Autodesk Fusion 360 part; units mm, degrees
note: some values were not read from the file. Set by a fixed rule: which sketch regions a step uses.
(part 18 of 59)
  spline S101 degree 5 poles (29.3284, 22.5421) (29.3257, 22.5422) (29.3203, 22.5423) (29.3122, 22.5425) (29.3014, 22.5428) (29.288, 22.5431) (29.2745, 22.5434) (29.2612, 22.5437) (29.2478, 22.544) (29.2345, 22.5442) (29.2212, 22.5445) (29.2079, 22.5447) (29.1947, 22.5449) (29.1815, 22.5451) (29.1683, 22.5453) (29.1551, 22.5454) (29.142, 22.5455) (29.129, 22.5457) (29.1159, 22.5458) (29.1029, 22.5458) (29.0899, 22.5459) (29.077, 22.546) (29.0641, 22.546) (29.0512, 22.546) (29.0383, 22.546) (29.0255, 22.546) (29.0127, 22.546) (29, 22.5459) (28.9872, 22.5458) (28.9745, 22.5458) (28.9619, 22.5457) (28.9493, 22.5456) (28.9367, 22.5454) (28.9241, 22.5453) (28.9116, 22.5451) (28.8991, 22.5449) (28.8867, 22.5448) (28.8743, 22.5445) (28.8619, 22.5443) (28.8495, 22.5441) (28.8372, 22.5438) (28.8249, 22.5436) (28.8127, 22.5433) (28.8005, 22.543) (28.7883, 22.5427) (28.7762, 22.5423) (28.7641, 22.542) (28.752, 22.5416) (28.74, 22.5412) (28.728, 22.5409) (28.716, 22.5405) (28.7041, 22.54) (28.6922, 22.5396) (28.6803, 22.5392) (28.6685, 22.5387) (28.6567, 22.5382) (28.645, 22.5377) (28.6333, 22.5372) (28.6216, 22.5367) (28.61, 22.5362) (28.5984, 22.5356) (28.5868, 22.5351) (28.5753, 22.5345) (28.5638, 22.5339) (28.5524, 22.5333) (28.541, 22.5327) (28.5296, 22.5321) (28.5183, 22.5314) (28.507, 22.5308) (28.4957, 22.5301) (28.4845, 22.5294) (28.4733, 22.5287) (28.4622, 22.528) (28.4511, 22.5273) (28.44, 22.5266) (28.429, 22.5258) (28.4181, 22.5251) (28.4071, 22.5243) (28.3962, 22.5235) (28.3854, 22.5227) (28.3745, 22.5219) (28.3638, 22.5211) (28.353, 22.5203) (28.3423, 22.5195) (28.3317, 22.5186) (28.321, 22.5177) (28.3105, 22.5169) (28.2999, 22.516) (28.2894, 22.5151) (28.279, 22.5142) (28.2686, 22.5133) (28.2582, 22.5123) (28.2479, 22.5114) (28.2376, 22.5104) (28.2274, 22.5095) (28.2172, 22.5085) (28.207, 22.5075) (28.1969, 22.5065) (28.1868, 22.5055) (28.1768, 22.5045) (28.1668, 22.5035) (28.1569, 22.5025) (28.147, 22.5014) (28.1372, 22.5004) (28.1274, 22.4993) (28.1176, 22.4983) (28.1079, 22.4972) (28.0982, 22.4961) (28.0886, 22.495) (28.079, 22.4939) (28.0695, 22.4928) (28.06, 22.4916) (28.0506, 22.4905) (28.0412, 22.4894) (28.0318, 22.4882) (28.0225, 22.4871) (28.0133, 22.4859) (28.004, 22.4847) (27.9949, 22.4836) (27.9858, 22.4824) (27.9767, 22.4812) (27.9677, 22.48) (27.9587, 22.4788) (27.9498, 22.4776) (27.9409, 22.4763) (27.9321, 22.4751) (27.9233, 22.4739) (27.9146, 22.4726) (27.9059, 22.4714) (27.8973, 22.4701) (27.8887, 22.4689) (27.8802, 22.4676) (27.8717, 22.4664) (27.8633, 22.4651) (27.8549, 22.4638) (27.8466, 22.4625) (27.8383, 22.4612) (27.8301, 22.4599) (27.8219, 22.4586) (27.8138, 22.4573) (27.8057, 22.456) (27.7977, 22.4547) (27.7898, 22.4534) (27.7819, 22.4521) (27.774, 22.4508) (27.7662, 22.4494) (27.7585, 22.4481) (27.7508, 22.4468) (27.7431, 22.4454) (27.7356, 22.4441) (27.728, 22.4428) (27.7206, 22.4414) (27.7132, 22.4401) (27.7058, 22.4387) (27.6985, 22.4374) (27.6912, 22.436) (27.6841, 22.4347) (27.6769, 22.4333) (27.6698, 22.432) (27.6628, 22.4306) (27.6559, 22.4293) (27.649, 22.4279) (27.6421, 22.4266) (27.6353, 22.4252) (27.6286, 22.4239) (27.622, 22.4225) (27.6154, 22.4212) (27.6088, 22.4199) (27.6023, 22.4185) (27.5959, 22.4172) (27.5896, 22.4158) (27.5833, 22.4145) (27.577, 22.4132) (27.5709, 22.4118) (27.5647, 22.4105) (27.5587, 22.4092) (27.5527, 22.4079) (27.5468, 22.4065) (27.5409, 22.4052) (27.5352, 22.4039) (27.5294, 22.4026) (27.5238, 22.4013) (27.5182, 22.4) (27.5127, 22.3987) (27.5072, 22.3974) (27.5018, 22.3962) (27.4965, 22.3949) (27.4912, 22.3936) (27.4861, 22.3924) (27.481, 22.3911) (27.4759, 22.3899) (27.4709, 22.3887) (27.466, 22.3874) (27.4612, 22.3862) (27.4564, 22.385) (27.4517, 22.3838) (27.4471, 22.3827) (27.4426, 22.3815) (27.4381, 22.3803) (27.4337, 22.3792) (27.4294, 22.378) (27.4252, 22.3769) (27.421, 22.3758) (27.4169, 22.3747) (27.4129, 22.3736) (27.409, 22.3725) (27.4051, 22.3715) (27.4013, 22.3704) (27.3976, 22.3694) (27.394, 22.3684) (27.3905, 22.3674) (27.387, 22.3664) (27.3837, 22.3654) (27.3804, 22.3645) (27.3772, 22.3635) (27.3741, 22.3626) (27.371, 22.3617) (27.3681, 22.3608) (27.3652, 22.36) (27.3625, 22.3591) (27.3598, 22.3583) (27.3572, 22.3575) (27.3547, 22.3568) (27.3523, 22.356) (27.3499, 22.3553) (27.3477, 22.3546) (27.3456, 22.3539) (27.3435, 22.3533) (27.3416, 22.3527) (27.3398, 22.3521) (27.338, 22.3515) (27.3364, 22.351) (27.3348, 22.3505) (27.3334, 22.35) (27.332, 22.3495) (27.3308, 22.3491) (27.3296, 22.3487) (27.3286, 22.3484) (27.3277, 22.3481) (27.3269, 22.3478) (27.3262, 22.3475) (27.3257, 22.3474) (27.3254, 22.3473) (27.3252, 22.3472) (27.3251, 22.3472) knots -1 -1 -1 -1 -1 -1 -0.99583333 -0.99166667 -0.9875 -0.98333333 -0.97916667 -0.975 -0.97083333 -0.96666667 -0.9625 -0.95833333 -0.95416667 -0.95 -0.94583333 -0.94166667 -0.9375 -0.93333333 -0.92916667 -0.925 -0.92083333 -0.91666667 -0.9125 -0.90833333 -0.90416667 -0.9 -0.89583333 -0.89166667 -0.8875 -0.88333333 -0.87916667 -0.875 -0.87083333 -0.86666667 -0.8625 -0.85833333 -0.85416667 -0.85 -0.84583333 -0.84166667 -0.8375 -0.83333333 -0.82916667 -0.825 -0.82083333 -0.81666667 -0.8125 -0.80833333 -0.80416667 -0.8 -0.79583333 -0.79166667 -0.7875 -0.78333333 -0.77916667 -0.775 -0.77083333 -0.76666667 -0.7625 -0.75833333 -0.75416667 -0.75 -0.74583333 -0.74166667 -0.7375 -0.73333333 -0.72916667 -0.725 -0.72083333 -0.71666667 -0.7125 -0.70833333 -0.70416667 -0.7 -0.69583333 -0.69166667 -0.6875 -0.68333333 -0.67916667 -0.675 -0.67083333 -0.66666667 -0.6625 -0.65833333 -0.65416667 -0.65 -0.64583333 -0.64166667 -0.6375 -0.63333333 -0.62916667 -0.625 -0.62083333 -0.61666667 -0.6125 -0.60833333 -0.60416667 -0.6 -0.59583333 -0.59166667 -0.5875 -0.58333333 -0.57916667 -0.575 -0.57083333 -0.56666667 -0.5625 -0.55833333 -0.55416667 -0.55 -0.54583333 -0.54166667 -0.5375 -0.53333333 -0.52916667 -0.525 -0.52083333 -0.51666667 -0.5125 -0.50833333 -0.50416667 -0.5 -0.49583333 -0.49166667 -0.4875 -0.48333333 -0.47916667 -0.475 -0.47083333 -0.46666667 -0.4625 -0.45833333 -0.45416667 -0.45 -0.44583333 -0.44166667 -0.4375 -0.43333333 -0.42916667 -0.425 -0.42083333 -0.41666667 -0.4125 -0.40833333 -0.40416667 -0.4 -0.39583333 -0.39166667 -0.3875 -0.38333333 -0.37916667 -0.375 -0.37083333 -0.36666667 -0.3625 -0.35833333 -0.35416667 -0.35 -0.34583333 -0.34166667 -0.3375 -0.33333333 -0.32916667 -0.325 -0.32083333 -0.31666667 -0.3125 -0.30833333 -0.30416667 -0.3 -0.29583333 -0.29166667 -0.2875 -0.28333333 -0.27916667 -0.275 -0.27083333 -0.26666667 -0.2625 -0.25833333 -0.25416667 -0.25 -0.24583333 -0.24166667 -0.2375 -0.23333333 -0.22916667 -0.225 -0.22083333 -0.21666667 -0.2125 -0.20833333 -0.20416667 -0.2 -0.19583333 -0.19166667 -0.1875 -0.18333333 -0.17916667 -0.175 -0.17083333 -0.16666667 -0.1625 -0.15833333 -0.15416667 -0.15 -0.14583333 -0.14166667 -0.1375 -0.13333333 -0.12916667 -0.125 -0.12083333 -0.11666667 -0.1125 -0.10833333 -0.10416667 -0.1 -0.09583333 -0.09166667 -0.0875 -0.08333333 -0.07916667 -0.075 -0.07083333 -0.06666667 -0.0625 -0.05833333 -0.05416667 -0.05 -0.04583333 -0.04166667 -0.0375 -0.03333333 -0.02916667 -0.025 -0.02083333 -0.01666667 -0.0125 -0.00833333 -0.00416667 0 0 0 0 0 0
  arc A109 (17.8246, -12.863) -> (18.6136, -12.2898) centre (0, 12.5) ccw
  line L228 (20.1094, -8.4569) -> (19.9055, -8.2445)
  arc A110 (20.7445, 32.4055) -> (19.9055, 33.2445) centre (0, 12.5) ccw
  arc A111 (-27.918, 5.6335) -> (-27.6109, 4.4875) centre (0, 12.5) ccw
  line L229 (-26.6221, 1.6453) -> (-26.8948, 1.5341)
  line L230 (20.1094, 33.4569) -> (20.11, 33.4575)
  line L231 (-27.3251, 2.6528) -> (-27.3243, 2.6531)
  arc A112 (-30.4202, 6.5325) -> (-30.2174, 5.5786) centre (0, 12.5) ccw
  spline S102 degree 5 poles (24.7898, 31.1136) (24.7872, 31.1128) (24.782, 31.1113) (24.7743, 31.109) (24.7639, 31.1059) (24.751, 31.1021) (24.7382, 31.0982) (24.7253, 31.0943) (24.7125, 31.0905) (24.6998, 31.0866) (24.6871, 31.0827) (24.6744, 31.0788) (24.6617, 31.0749) (24.6491, 31.071) (24.6365, 31.0671) (24.624, 31.0632) (24.6115, 31.0593) (24.599, 31.0553) (24.5866, 31.0514) (24.5742, 31.0475) (24.5618, 31.0435) (24.5495, 31.0395) (24.5372, 31.0356) (24.5249, 31.0316) (24.5127, 31.0277) (24.5005, 31.0237) (24.4884, 31.0197) (24.4762, 31.0157) (24.4642, 31.0117) (24.4521, 31.0077) (24.4401, 31.0037) (24.4281, 30.9997) (24.4162, 30.9957) (24.4043, 30.9917) (24.3925, 30.9877) (24.3806, 30.9836) (24.3689, 30.9796) (24.3571, 30.9756) (24.3454, 30.9715) (24.3337, 30.9675) (24.3221, 30.9634) (24.3105, 30.9594) (24.299, 30.9553) (24.2874, 30.9513) (24.276, 30.9472) (24.2645, 30.9431) (24.2531, 30.9391) (24.2417, 30.935) (24.2304, 30.9309) (24.2191, 30.9269) (24.2079, 30.9228) (24.1967, 30.9187) (24.1855, 30.9146) (24.1744, 30.9105) (24.1633, 30.9064) (24.1522, 30.9023) (24.1412, 30.8982) (24.1302, 30.8941) (24.1193, 30.89) (24.1084, 30.8859) (24.0975, 30.8818) (24.0867, 30.8777) (24.0759, 30.8736) (24.0652, 30.8695) (24.0545, 30.8654) (24.0438, 30.8613) (24.0332, 30.8572) (24.0226, 30.8531) (24.0121, 30.849) (24.0016, 30.8449) (23.9911, 30.8408) (23.9807, 30.8366) (23.9703, 30.8325) (23.96, 30.8284) (23.9497, 30.8243) (23.9395, 30.8202) (23.9292, 30.8161) (23.9191, 30.812) (23.909, 30.8079) (23.8989, 30.8038) (23.8888, 30.7996) (23.8788, 30.7955) (23.8689, 30.7914) (23.859, 30.7873) (23.8491, 30.7832) (23.8393, 30.7791) (23.8295, 30.775) (23.8197, 30.7709) (23.81, 30.7668) (23.8004, 30.7627) (23.7907, 30.7587) (23.7812, 30.7546) (23.7716, 30.7505) (23.7622, 30.7464) (23.7527, 30.7423) (23.7433, 30.7383) (23.734, 30.7342) (23.7247, 30.7301) (23.7154, 30.726) (23.7062, 30.722) (23.697, 30.7179) (23.6879, 30.7139) (23.6788, 30.7098) (23.6697, 30.7058) (23.6607, 30.7018) (23.6518, 30.6977) (23.6429, 30.6937) (23.634, 30.6897) (23.6252, 30.6857) (23.6165, 30.6816) (23.6077, 30.6776) (23.5991, 30.6736) (23.5904, 30.6696) (23.5818, 30.6657) (23.5733, 30.6617) (23.5648, 30.6577) (23.5564, 30.6537) (23.548, 30.6498) (23.5396, 30.6458) (23.5313, 30.6419) (23.5231, 30.6379) (23.5149, 30.634) (23.5067, 30.6301) (23.4986, 30.6262) (23.4905, 30.6223) (23.4825, 30.6184) (23.4746, 30.6145) (23.4666, 30.6106) (23.4588, 30.6068) (23.451, 30.6029) (23.4432, 30.5991) (23.4355, 30.5952) (23.4278, 30.5914) (23.4202, 30.5876) (23.4126, 30.5838) (23.4051, 30.58) (23.3976, 30.5762) (23.3902, 30.5724) (23.3828, 30.5687) (23.3755, 30.5649) (23.3683, 30.5612) (23.361, 30.5575) (23.3539, 30.5538) (23.3468, 30.5501) (23.3397, 30.5464) (23.3327, 30.5427) (23.3257, 30.539) (23.3188, 30.5354) (23.312, 30.5318) (23.3052, 30.5282) (23.2984, 30.5246) (23.2918, 30.521) (23.2851, 30.5174) (23.2785, 30.5139) (23.272, 30.5103) (23.2655, 30.5068) (23.2591, 30.5033) (23.2527, 30.4998) (23.2464, 30.4963) (23.2402, 30.4929) (23.234, 30.4895) (23.2278, 30.486) (23.2217, 30.4826) (23.2157, 30.4793) (23.2097, 30.4759) (23.2038, 30.4726) (23.1979, 30.4692) (23.1921, 30.4659) (23.1864, 30.4627) (23.1807, 30.4594) (23.1751, 30.4562) (23.1695, 30.4529) (23.164, 30.4497) (23.1585, 30.4466) (23.1531, 30.4434) (23.1478, 30.4403) (23.1425, 30.4372) (23.1373, 30.4341) (23.1321, 30.431) (23.127, 30.428) (23.122, 30.425) (23.117, 30.422) (23.1121, 30.4191) (23.1072, 30.4161) (23.1024, 30.4132) (23.0977, 30.4103) (23.093, 30.4075) (23.0884, 30.4047) (23.0839, 30.4019) (23.0794, 30.3991) (23.075, 30.3964) (23.0706, 30.3937) (23.0664, 30.391) (23.0621, 30.3883) (23.058, 30.3857) (23.0539, 30.3831) (23.0499, 30.3806) (23.0459, 30.3781) (23.042, 30.3756) (23.0382, 30.3731) (23.0344, 30.3707) (23.0308, 30.3683) (23.0271, 30.366) (23.0236, 30.3637) (23.0201, 30.3614) (23.0167, 30.3592) (23.0134, 30.357) (23.0101, 30.3548) (23.0069, 30.3527) (23.0038, 30.3506) (23.0007, 30.3485) (22.9978, 30.3465) (22.9948, 30.3446) (22.992, 30.3427) (22.9893, 30.3408) (22.9866, 30.3389) (22.984, 30.3372) (22.9814, 30.3354) (22.979, 30.3337) (22.9766, 30.3321) (22.9743, 30.3305) (22.9721, 30.3289) (22.9699, 30.3274) (22.9679, 30.326) (22.9659, 30.3246) (22.964, 30.3232) (22.9622, 30.3219) (22.9604, 30.3207) (22.9588, 30.3195) (22.9572, 30.3183) (22.9557, 30.3172) (22.9543, 30.3162) (22.953, 30.3153) (22.9518, 30.3144) (22.9506, 30.3135) (22.9496, 30.3127) (22.9486, 30.312) (22.9477, 30.3114) (22.9469, 30.3108) (22.9463, 30.3103) (22.9457, 30.3098) (22.9453, 30.3095) (22.945, 30.3093) (22.9448, 30.3092) (22.9448, 30.3091) knots -1 -1 -1 -1 -1 -1 -0.99583333 -0.99166667 -0.9875 -0.98333333 -0.97916667 -0.975 -0.97083333 -0.96666667 -0.9625 -0.95833333 -0.95416667 -0.95 -0.94583333 -0.94166667 -0.9375 -0.93333333 -0.92916667 -0.925 -0.92083333 -0.91666667 -0.9125 -0.90833333 -0.90416667 -0.9 -0.89583333 -0.89166667 -0.8875 -0.88333333 -0.87916667 -0.875 -0.87083333 -0.86666667 -0.8625 -0.85833333 -0.85416667 -0.85 -0.84583333 -0.84166667 -0.8375 -0.83333333 -0.82916667 -0.825 -0.82083333 -0.81666667 -0.8125 -0.80833333 -0.80416667 -0.8 -0.79583333 -0.79166667 -0.7875 -0.78333333 -0.77916667 -0.775 -0.77083333 -0.76666667 -0.7625 -0.75833333 -0.75416667 -0.75 -0.74583333 -0.74166667 -0.7375 -0.73333333 -0.72916667 -0.725 -0.72083333 -0.71666667 -0.7125 -0.70833333 -0.70416667 -0.7 -0.69583333 -0.69166667 -0.6875 -0.68333333 -0.67916667 -0.675 -0.67083333 -0.66666667 -0.6625 -0.65833333 -0.65416667 -0.65 -0.64583333 -0.64166667 -0.6375 -0.63333333 -0.62916667 -0.625 -0.62083333 -0.61666667 -0.6125 -0.60833333 -0.60416667 -0.6 -0.59583333 -0.59166667 -0.5875 -0.58333333 -0.57916667 -0.575 -0.57083333 -0.56666667 -0.5625 -0.55833333 -0.55416667 -0.55 -0.54583333 -0.54166667 -0.5375 -0.53333333 -0.52916667 -0.525 -0.52083333 -0.51666667 -0.5125 -0.50833333 -0.50416667 -0.5 -0.49583333 -0.49166667 -0.4875 -0.48333333 -0.47916667 -0.475 -0.47083333 -0.46666667 -0.4625 -0.45833333 -0.45416667 -0.45 -0.44583333 -0.44166667 -0.4375 -0.43333333 -0.42916667 -0.425 -0.42083333 -0.41666667 -0.4125 -0.40833333 -0.40416667 -0.4 -0.39583333 -0.39166667 -0.3875 -0.38333333 -0.37916667 -0.375 -0.37083333 -0.36666667 -0.3625 -0.35833333 -0.35416667 -0.35 -0.34583333 -0.34166667 -0.3375 -0.33333333 -0.32916667 -0.325 -0.32083333 -0.31666667 -0.3125 -0.30833333 -0.30416667 -0.3 -0.29583333 -0.29166667 -0.2875 -0.28333333 -0.27916667 -0.275 -0.27083333 -0.26666667 -0.2625 -0.25833333 -0.25416667 -0.25 -0.24583333 -0.24166667 -0.2375 -0.23333333 -0.22916667 -0.225 -0.22083333 -0.21666667 -0.2125 -0.20833333 -0.20416667 -0.2 -0.19583333 -0.19166667 -0.1875 -0.18333333 -0.17916667 -0.175 -0.17083333 -0.16666667 -0.1625 -0.15833333 -0.15416667 -0.15 -0.14583333 -0.14166667 -0.1375 -0.13333333 -0.12916667 -0.125 -0.12083333 -0.11666667 -0.1125 -0.10833333 -0.10416667 -0.1 -0.09583333 -0.09166667 -0.0875 -0.08333333 -0.07916667 -0.075 -0.07083333 -0.06666667 -0.0625 -0.05833333 -0.05416667 -0.05 -0.04583333 -0.04166667 -0.0375 -0.03333333 -0.02916667 -0.025 -0.02083333 -0.01666667 -0.0125 -0.00833333 -0.00416667 0 0 0 0 0 0
  arc A113 (-27.0473, 2.7529) -> (-26.6221, 1.6453) centre (0, 12.5) ccw
  spline S103 degree 5 poles (24.0278, 28.8184) (24.0279, 28.8185) (24.0281, 28.8186) (24.0283, 28.8188) (24.0287, 28.8191) (24.0294, 28.8195) (24.0301, 28.82) (24.0309, 28.8206) (24.0317, 28.8212) (24.0327, 28.8219) (24.0338, 28.8227) (24.035, 28.8235) (24.0362, 28.8244) (24.0375, 28.8253) (24.0389, 28.8263) (24.0404, 28.8274) (24.042, 28.8286) (24.0436, 28.8298) (24.0453, 28.831) (24.0471, 28.8324) (24.049, 28.8338) (24.051, 28.8352) (24.053, 28.8367) (24.0551, 28.8383) (24.0572, 28.8399) (24.0595, 28.8416) (24.0618, 28.8434) (24.0641, 28.8452) (24.0666, 28.8471) (24.0691, 28.849) (24.0717, 28.851) (24.0743, 28.853) (24.077, 28.8551) (24.0798, 28.8573) (24.0826, 28.8595) (24.0855, 28.8618) (24.0884, 28.8641) (24.0914, 28.8665) (24.0945, 28.8689) (24.0976, 28.8714) (24.1008, 28.874) (24.104, 28.8766) (24.1073, 28.8792) (24.1107, 28.8819) (24.1141, 28.8847) (24.1176, 28.8875) (24.1211, 28.8904) (24.1246, 28.8933) (24.1283, 28.8963) (24.1319, 28.8994) (24.1356, 28.9024) (24.1394, 28.9056) (24.1432, 28.9088) (24.1471, 28.912) (24.151, 28.9153) (24.155, 28.9187) (24.159, 28.9221) (24.1631, 28.9256) (24.1672, 28.9291) (24.1713, 28.9326) (24.1755, 28.9362) (24.1798, 28.9399) (24.1841, 28.9436) (24.1884, 28.9474) (24.1928, 28.9512) (24.1972, 28.955) (24.2017, 28.959) (24.2062, 28.9629) (24.2107, 28.9669) (24.2153, 28.971) (24.2199, 28.9751) (24.2246, 28.9793) (24.2293, 28.9835) (24.234, 28.9877) (24.2388, 28.992) (24.2436, 28.9964) (24.2485, 29.0008) (24.2534, 29.0053) (24.2583, 29.0098) (24.2633, 29.0143) (24.2683, 29.0189) (24.2733, 29.0236) (24.2784, 29.0282) (24.2835, 29.033) (24.2887, 29.0378) (24.2939, 29.0426) (24.2991, 29.0475) (24.3043, 29.0524) (24.3096, 29.0574) (24.3149, 29.0624) (24.3203, 29.0675) (24.3257, 29.0726) (24.3311, 29.0778) (24.3365, 29.083) (24.342, 29.0882) (24.3475, 29.0935) (24.353, 29.0989) (24.3586, 29.1043) (24.3642, 29.1097) (24.3698, 29.1152) (24.3755, 29.1207) (24.3812, 29.1263) (24.3869, 29.1319) (24.3926, 29.1376) (24.3984, 29.1433) (24.4042, 29.1491) (24.41, 29.1549) (24.4159, 29.1607) (24.4218, 29.1666) (24.4277, 29.1725) (24.4336, 29.1785) (24.4395, 29.1845) (24.4455, 29.1906) (24.4515, 29.1967) (24.4576, 29.2029) (24.4636, 29.2091) (24.4697, 29.2153) (24.4758, 29.2216) (24.482, 29.2279) (24.4881, 29.2343) (24.4943, 29.2407) (24.5005, 29.2472) (24.5067, 29.2537) (24.513, 29.2602) (24.5192, 29.2668) (24.5255, 29.2735) (24.5319, 29.2801) (24.5382, 29.2869) (24.5446, 29.2936) (24.5509, 29.3004) (24.5573, 29.3073) (24.5638, 29.3142) (24.5702, 29.3211) (24.5767, 29.3281) (24.5831, 29.3351) (24.5897, 29.3421) (24.5962, 29.3492) (24.6027, 29.3564) (24.6093, 29.3636) (24.6159, 29.3708) (24.6225, 29.3781) (24.6291, 29.3854) (24.6357, 29.3927) (24.6424, 29.4001) (24.6491, 29.4075) (24.6558, 29.415) (24.6625, 29.4225) (24.6692, 29.4301) (24.6759, 29.4377) (24.6827, 29.4453) (24.6895, 29.453) (24.6963, 29.4607) (24.7031, 29.4685) (24.7099, 29.4763) (24.7168, 29.4841) (24.7236, 29.492) (24.7305, 29.4999) (24.7374, 29.5079) (24.7443, 29.5159) (24.7512, 29.5239) (24.7582, 29.532) (24.7651, 29.5401) (24.7721, 29.5483) (24.7791, 29.5565) (24.7861, 29.5647) (24.7931, 29.573) (24.8001, 29.5813) (24.8071, 29.5897) (24.8142, 29.5981) (24.8212, 29.6065) (24.8283, 29.615) (24.8354, 29.6235) (24.8425, 29.6321) (24.8496, 29.6407) (24.8568, 29.6493) (24.8639, 29.658) (24.8711, 29.6667) (24.8782, 29.6754) (24.8854, 29.6842) (24.8926, 29.6931) (24.8998, 29.7019) (24.907, 29.7108) (24.9142, 29.7198) (24.9215, 29.7288) (24.9287, 29.7378) (24.936, 29.7469) (24.9432, 29.7559) (24.9505, 29.7651) (24.9578, 29.7743) (24.9651, 29.7835) (24.9724, 29.7927) (24.9797, 29.802) (24.9871, 29.8113) (24.9944, 29.8207) (25.0017, 29.8301) (25.0091, 29.8395) (25.0165, 29.849) (25.0238, 29.8585) (25.0312, 29.8681) (25.0386, 29.8777) (25.046, 29.8873) (25.0534, 29.897) (25.0609, 29.9067) (25.0683, 29.9164) (25.0757, 29.9262) (25.0832, 29.936) (25.0906, 29.9458) (25.0981, 29.9557) (25.1055, 29.9657) (25.113, 29.9756) (25.1205, 29.9856) (25.128, 29.9956) (25.1355, 30.0057) (25.143, 30.0158) (25.1505, 30.026) (25.158, 30.0361) (25.1655, 30.0464) (25.1731, 30.0566) (25.1806, 30.0669) (25.1881, 30.0772) (25.1957, 30.0876) (25.2032, 30.098) (25.2108, 30.1084) (25.2184, 30.1189) (25.2259, 30.1294) (25.2335, 30.1399) (25.2411, 30.1505) (25.2487, 30.1611) (25.2563, 30.1718) (25.2639, 30.1825) (25.2715, 30.1932) (25.2791, 30.2039) (25.2867, 30.2147) (25.2943, 30.2256) (25.3019, 30.2364) (25.3096, 30.2473) (25.3172, 30.2583) (25.3248, 30.2692) (25.3325, 30.2802) (25.3401, 30.2913) (25.3477, 30.3023) (25.3539, 30.3112) (25.3584, 30.3179) (25.3615, 30.3224) (25.363, 30.3246) knots 0 0 0 0 0 0 0.00416667 0.00833333 0.0125 0.01666667 0.02083333 0.025 0.02916667 0.03333333 0.0375 0.04166667 0.04583333 0.05 0.05416667 0.05833333 0.0625 0.06666667 0.07083333 0.075 0.07916667 0.08333333 0.0875 0.09166667 0.09583333 0.1 0.10416667 0.10833333 0.1125 0.11666667 0.12083333 0.125 0.12916667 0.13333333 0.1375 0.14166667 0.14583333 0.15 0.15416667 0.15833333 0.1625 0.16666667 0.17083333 0.175 0.17916667 0.18333333 0.1875 0.19166667 0.19583333 0.2 0.20416667 0.20833333 0.2125 0.21666667 0.22083333 0.225 0.22916667 0.23333333 0.2375 0.24166667 0.24583333 0.25 0.25416667 0.25833333 0.2625 0.26666667 0.27083333 0.275 0.27916667 0.28333333 0.2875 0.29166667 0.29583333 0.3 0.30416667 0.30833333 0.3125 0.31666667 0.32083333 0.325 0.32916667 0.33333333 0.3375 0.34166667 0.34583333 0.35 0.35416667 0.35833333 0.3625 0.36666667 0.37083333 0.375 0.37916667 0.38333333 0.3875 0.39166667 0.39583333 0.4 0.40416667 0.40833333 0.4125 0.41666667 0.42083333 0.425 0.42916667 0.43333333 0.4375 0.44166667 0.44583333 0.45 0.45416667 0.45833333 0.4625 0.46666667 0.47083333 0.475 0.47916667 0.48333333 0.4875 0.49166667 0.49583333 0.5 0.50416667 0.50833333 0.5125 0.51666667 0.52083333 0.525 0.52916667 0.53333333 0.5375 0.54166667 0.54583333 0.55 0.55416667 0.55833333 0.5625 0.56666667 0.57083333 0.575 0.57916667 0.58333333 0.5875 0.59166667 0.59583333 0.6 0.60416667 0.60833333 0.6125 0.61666667 0.62083333 0.625 0.62916667 0.63333333 0.6375 0.64166667 0.64583333 0.65 0.65416667 0.65833333 0.6625 0.66666667 0.67083333 0.675 0.67916667 0.68333333 0.6875 0.69166667 0.69583333 0.7 0.70416667 0.70833333 0.7125 0.71666667 0.72083333 0.725 0.72916667 0.73333333 0.7375 0.74166667 0.74583333 0.75 0.75416667 0.75833333 0.7625 0.76666667 0.77083333 0.775 0.77916667 0.78333333 0.7875 0.79166667 0.79583333 0.8 0.80416667 0.80833333 0.8125 0.81666667 0.82083333 0.825 0.82916667 0.83333333 0.8375 0.84166667 0.84583333 0.85 0.85416667 0.85833333 0.8625 0.86666667 0.87083333 0.875 0.87916667 0.88333333 0.8875 0.89166667 0.89583333 0.9 0.90416667 0.90833333 0.9125 0.91666667 0.92083333 0.925 0.92916667 0.93333333 0.9375 0.94166667 0.94583333 0.95 0.95416667 0.95833333 0.9625 0.96666667 0.97083333 0.975 0.97916667 0.98333333 0.9875 0.99166667 0.99583333 1 1 1 1 1 1
  arc A114 (22.7115, 30.1281) -> (21.9649, 31.0501) centre (0, 12.5) ccw
  arc A115 (21.1029, 35.2084) -> (20.3781, 35.8609) centre (0, 12.5) ccw
  spline S104 degree 5 poles (-12.1618, -16.0147) (-12.16, -16.0128) (-12.1562, -16.0089) (-12.1506, -16.003) (-12.1432, -15.9951) (-12.134, -15.9854) (-12.1248, -15.9756) (-12.1156, -15.9658) (-12.1065, -15.9561) (-12.0973, -15.9464) (-12.0883, -15.9366) (-12.0792, -15.9269) (-12.0702, -15.9172) (-12.0613, -15.9075) (-12.0523, -15.8978) (-12.0434, -15.8882) (-12.0345, -15.8785) (-12.0257, -15.8689) (-12.0169, -15.8593) (-12.0081, -15.8496) (-11.9994, -15.84) (-11.9907, -15.8305) (-11.982, -15.8209) (-11.9734, -15.8113) (-11.9648, -15.8018) (-11.9562, -15.7922) (-11.9477, -15.7827) (-11.9392, -15.7732) (-11.9307, -15.7637) (-11.9223, -15.7542) (-11.9139, -15.7447) (-11.9055, -15.7353) (-11.8972, -15.7259) (-11.8889, -15.7164) (-11.8807, -15.707) (-11.8724, -15.6976) (-11.8643, -15.6882) (-11.8561, -15.6789) (-11.848, -15.6695) (-11.8399, -15.6602) (-11.8318, -15.6509) (-11.8238, -15.6416) (-11.8158, -15.6323) (-11.8079, -15.623) (-11.8, -15.6137) (-11.7921, -15.6045) (-11.7843, -15.5953) (-11.7765, -15.5861) (-11.7687, -15.5769) (-11.7609, -15.5677) (-11.7532, -15.5585) (-11.7456, -15.5494) (-11.7379, -15.5403) (-11.7303, -15.5312) (-11.7228, -15.5221) (-11.7153, -15.513) (-11.7078, -15.5039) (-11.7003, -15.4949) (-11.6929, -15.4859) (-11.6855, -15.4769) (-11.6781, -15.4679) (-11.6708, -15.4589) (-11.6635, -15.45) (-11.6563, -15.4411) (-11.6491, -15.4322) (-11.6419, -15.4233) (-11.6348, -15.4144) (-11.6276, -15.4055) (-11.6206, -15.3967) (-11.6135, -15.3879) (-11.6065, -15.3791) (-11.5996, -15.3704) (-11.5927, -15.3616) (-11.5858, -15.3529) (-11.5789, -15.3442) (-11.5721, -15.3355) (-11.5653, -15.3268) (-11.5585, -15.3182) (-11.5518, -15.3096) (-11.5452, -15.301) (-11.5385, -15.2924) (-11.5319, -15.2838) (-11.5253, -15.2753) (-11.5188, -15.2668) (-11.5123, -15.2583) (-11.5058, -15.2498) (-11.4994, -15.2414) (-11.493, -15.233) (-11.4867, -15.2246) (-11.4803, -15.2162) (-11.4741, -15.2078) (-11.4678, -15.1995) (-11.4616, -15.1912) (-11.4554, -15.1829) (-11.4493, -15.1747) (-11.4432, -15.1665) (-11.4371, -15.1582) (-11.4311, -15.1501) (-11.4251, -15.1419) (-11.4192, -15.1338) (-11.4132, -15.1257) (-11.4074, -15.1176) (-11.4015, -15.1096) (-11.3957, -15.1015) (-11.3899, -15.0936) (-11.3842, -15.0856) (-11.3785, -15.0776) (-11.3728, -15.0697) (-11.3672, -15.0618) (-11.3616, -15.054) (-11.3561, -15.0462) (-11.3506, -15.0384) (-11.3451, -15.0306) (-11.3396, -15.0228) (-11.3342, -15.0151) (-11.3289, -15.0074) (-11.3235, -14.9998) (-11.3183, -14.9922) (-11.313, -14.9846) (-11.3078, -14.977) (-11.3026, -14.9695) (-11.2975, -14.962) (-11.2924, -14.9545) (-11.2873, -14.947) (-11.2823, -14.9396) (-11.2773, -14.9323) (-11.2723, -14.9249) (-11.2674, -14.9176) (-11.2625, -14.9103) (-11.2577, -14.9031) (-11.2529, -14.8958) (-11.2481, -14.8887) (-11.2434, -14.8815) (-11.2387, -14.8744) (-11.234, -14.8673) (-11.2294, -14.8603) (-11.2248, -14.8533) (-11.2203, -14.8463) (-11.2158, -14.8393) (-11.2113, -14.8324) (-11.2069, -14.8256) (-11.2025, -14.8187) (-11.1982, -14.8119) (-11.1939, -14.8052) (-11.1896, -14.7985) (-11.1854, -14.7918) (-11.1812, -14.7851) (-11.177, -14.7785) (-11.1729, -14.772) (-11.1688, -14.7654) (-11.1648, -14.759) (-11.1608, -14.7525) (-11.1568, -14.7461) (-11.1529, -14.7397) (-11.149, -14.7334) (-11.1451, -14.7271) (-11.1413, -14.7209) (-11.1376, -14.7147) (-11.1338, -14.7085) (-11.1301, -14.7024) (-11.1265, -14.6963) (-11.1229, -14.6903) (-11.1193, -14.6843) (-11.1158, -14.6784) (-11.1123, -14.6725) (-11.1088, -14.6666) (-11.1054, -14.6608) (-11.102, -14.655) (-11.0987, -14.6493) (-11.0954, -14.6436) (-11.0921, -14.638) (-11.0889, -14.6324) (-11.0857, -14.6269) (-11.0826, -14.6214) (-11.0795, -14.616) (-11.0764, -14.6106) (-11.0734, -14.6053) (-11.0704, -14.6) (-11.0675, -14.5948) (-11.0646, -14.5896) (-11.0617, -14.5845) (-11.0589, -14.5794) (-11.0561, -14.5744) (-11.0534, -14.5694) (-11.0507, -14.5645) (-11.048, -14.5597) (-11.0454, -14.5549) (-11.0428, -14.5501) (-11.0403, -14.5454) (-11.0378, -14.5408) (-11.0353, -14.5362) (-11.0329, -14.5317) (-11.0306, -14.5272) (-11.0282, -14.5228) (-11.0259, -14.5185) (-11.0237, -14.5142) (-11.0215, -14.51) (-11.0193, -14.5058) (-11.0172, -14.5017) (-11.0151, -14.4977) (-11.0131, -14.4937) (-11.0111, -14.4898) (-11.0091, -14.486) (-11.0072, -14.4822) (-11.0053, -14.4785) (-11.0035, -14.4748) (-11.0017, -14.4713) (-10.9999, -14.4678) (-10.9982, -14.4643) (-10.9966, -14.461) (-10.9949, -14.4577) (-10.9934, -14.4544) (-10.9918, -14.4513) (-10.9903, -14.4482) (-10.9889, -14.4452) (-10.9875, -14.4423) (-10.9861, -14.4394) (-10.9848, -14.4366) (-10.9835, -14.4339) (-10.9823, -14.4313) (-10.9811, -14.4288) (-10.9799, -14.4263) (-10.9788, -14.424) (-10.9778, -14.4217) (-10.9768, -14.4195) (-10.9758, -14.4173) (-10.9749, -14.4153) (-10.974, -14.4134) (-10.9731, -14.4115) (-10.9724, -14.4097) (-10.9716, -14.408) (-10.9709, -14.4065) (-10.9702, -14.405) (-10.9696, -14.4036) (-10.9691, -14.4023) (-10.9685, -14.4011) (-10.9681, -14.4) (-10.9676, -14.399) (-10.9672, -14.3981) (-10.9669, -14.3973) (-10.9666, -14.3966) (-10.9664, -14.3961) (-10.9663, -14.3958) (-10.9662, -14.3956) (-10.9662, -14.3955) knots -1 -1 -1 -1 -1 -1 -0.99583333 -0.99166667 -0.9875 -0.98333333 -0.97916667 -0.975 -0.97083333 -0.96666667 -0.9625 -0.95833333 -0.95416667 -0.95 -0.94583333 -0.94166667 -0.9375 -0.93333333 -0.92916667 -0.925 -0.92083333 -0.91666667 -0.9125 -0.90833333 -0.90416667 -0.9 -0.89583333 -0.89166667 -0.8875 -0.88333333 -0.87916667 -0.875 -0.87083333 -0.86666667 -0.8625 -0.85833333 -0.85416667 -0.85 -0.84583333 -0.84166667 -0.8375 -0.83333333 -0.82916667 -0.825 -0.82083333 -0.81666667 -0.8125 -0.80833333 -0.80416667 -0.8 -0.79583333 -0.79166667 -0.7875 -0.78333333 -0.77916667 -0.775 -0.77083333 -0.76666667 -0.7625 -0.75833333 -0.75416667 -0.75 -0.74583333 -0.74166667 -0.7375 -0.73333333 -0.72916667 -0.725 -0.72083333 -0.71666667 -0.7125 -0.70833333 -0.70416667 -0.7 -0.69583333 -0.69166667 -0.6875 -0.68333333 -0.67916667 -0.675 -0.67083333 -0.66666667 -0.6625 -0.65833333 -0.65416667 -0.65 -0.64583333 -0.64166667 -0.6375 -0.63333333 -0.62916667 -0.625 -0.62083333 -0.61666667 -0.6125 -0.60833333 -0.60416667 -0.6 -0.59583333 -0.59166667 -0.5875 -0.58333333 -0.57916667 -0.575 -0.57083333 -0.56666667 -0.5625 -0.55833333 -0.55416667 -0.55 -0.54583333 -0.54166667 -0.5375 -0.53333333 -0.52916667 -0.525 -0.52083333 -0.51666667 -0.5125 -0.50833333 -0.50416667 -0.5 -0.49583333 -0.49166667 -0.4875 -0.48333333 -0.47916667 -0.475 -0.47083333 -0.46666667 -0.4625 -0.45833333 -0.45416667 -0.45 -0.44583333 -0.44166667 -0.4375 -0.43333333 -0.42916667 -0.425 -0.42083333 -0.41666667 -0.4125 -0.40833333 -0.40416667 -0.4 -0.39583333 -0.39166667 -0.3875 -0.38333333 -0.37916667 -0.375 -0.37083333 -0.36666667 -0.3625 -0.35833333 -0.35416667 -0.35 -0.34583333 -0.34166667 -0.3375 -0.33333333 -0.32916667 -0.325 -0.32083333 -0.31666667 -0.3125 -0.30833333 -0.30416667 -0.3 -0.29583333 -0.29166667 -0.2875 -0.28333333 -0.27916667 -0.275 -0.27083333 -0.26666667 -0.2625 -0.25833333 -0.25416667 -0.25 -0.24583333 -0.24166667 -0.2375 -0.23333333 -0.22916667 -0.225 -0.22083333 -0.21666667 -0.2125 -0.20833333 -0.20416667 -0.2 -0.19583333 -0.19166667 -0.1875 -0.18333333 -0.17916667 -0.175 -0.17083333 -0.16666667 -0.1625 -0.15833333 -0.15416667 -0.15 -0.14583333 -0.14166667 -0.1375 -0.13333333 -0.12916667 -0.125 -0.12083333 -0.11666667 -0.1125 -0.10833333 -0.10416667 -0.1 -0.09583333 -0.09166667 -0.0875 -0.08333333 -0.07916667 -0.075 -0.07083333 -0.06666667 -0.0625 -0.05833333 -0.05416667 -0.05 -0.04583333 -0.04166667 -0.0375 -0.03333333 -0.02916667 -0.025 -0.02083333 -0.01666667 -0.0125 -0.00833333 -0.00416667 0 0 0 0 0 0
  line L232 (-18.7406, -9.6904) -> (-18.7401, -9.6898)
  arc A116 (25.363, 30.3246) -> (24.7898, 31.1136) centre (0, 12.5) ccw
  line L233 (-18.7401, -9.6898) -> (-18.5501, -9.4649)
  line L234 (-29.0298, 13.4213) -> (-29.0307, 13.4213)
  spline S105 degree 5 poles (-28.2047, 19.437) (-28.2048, 19.437) (-28.205, 19.437) (-28.2053, 19.4371) (-28.2058, 19.4372) (-28.2065, 19.4374) (-28.2074, 19.4376) (-28.2083, 19.4378) (-28.2094, 19.4381) (-28.2106, 19.4383) (-28.2118, 19.4386) (-28.2132, 19.4389) (-28.2147, 19.4392) (-28.2163, 19.4396) (-28.218, 19.4399) (-28.2198, 19.4403) (-28.2217, 19.4407) (-28.2237, 19.4411) (-28.2258, 19.4416) (-28.228, 19.442) (-28.2303, 19.4425) (-28.2327, 19.4429) (-28.2351, 19.4434) (-28.2377, 19.4439) (-28.2404, 19.4445) (-28.2431, 19.445) (-28.246, 19.4455) (-28.2489, 19.4461) (-28.2519, 19.4466) (-28.255, 19.4472) (-28.2582, 19.4478) (-28.2615, 19.4484) (-28.2649, 19.449) (-28.2683, 19.4496) (-28.2719, 19.4502) (-28.2755, 19.4508) (-28.2792, 19.4515) (-28.283, 19.4521) (-28.2868, 19.4528) (-28.2908, 19.4534) (-28.2948, 19.4541) (-28.2989, 19.4547) (-28.3031, 19.4554) (-28.3074, 19.4561) (-28.3117, 19.4568) (-28.3161, 19.4574) (-28.3206, 19.4581) (-28.3252, 19.4588) (-28.3298, 19.4595) (-28.3345, 19.4602) (-28.3393, 19.4609) (-28.3442, 19.4616) (-28.3491, 19.4623) (-28.3541, 19.463) (-28.3592, 19.4637) (-28.3643, 19.4644) (-28.3695, 19.4651) (-28.3748, 19.4658) (-28.3802, 19.4665) (-28.3856, 19.4672) (-28.3911, 19.4679) (-28.3966, 19.4686) (-28.4023, 19.4693) (-28.408, 19.47) (-28.4137, 19.4707) (-28.4196, 19.4714) (-28.4255, 19.4721) (-28.4314, 19.4728) (-28.4374, 19.4735) (-28.4435, 19.4742) (-28.4497, 19.4749) (-28.4559, 19.4756) (-28.4622, 19.4763) (-28.4685, 19.4769) (-28.4749, 19.4776) (-28.4814, 19.4783) (-28.4879, 19.4789) (-28.4945, 19.4796) (-28.5011, 19.4803) (-28.5078, 19.4809) (-28.5146, 19.4816) (-28.5214, 19.4822) (-28.5283, 19.4828) (-28.5353, 19.4835) (-28.5423, 19.4841) (-28.5493, 19.4847) (-28.5564, 19.4853) (-28.5636, 19.4859) (-28.5709, 19.4865) (-28.5781, 19.4871) (-28.5855, 19.4877) (-28.5929, 19.4882) (-28.6004, 19.4888) (-28.6079, 19.4894) (-28.6154, 19.4899) (-28.6231, 19.4905) (-28.6307, 19.491) (-28.6385, 19.4915) (-28.6463, 19.4921) (-28.6541, 19.4926) (-28.662, 19.4931) (-28.67, 19.4936) (-28.678, 19.494) (-28.686, 19.4945) (-28.6941, 19.495) (-28.7023, 19.4954) (-28.7105, 19.4959) (-28.7187, 19.4963) (-28.727, 19.4968) (-28.7354, 19.4972) (-28.7438, 19.4976) (-28.7523, 19.498) (-28.7608, 19.4984) (-28.7694, 19.4987) (-28.778, 19.4991) (-28.7866, 19.4995) (-28.7953, 19.4998) (-28.8041, 19.5001) (-28.8129, 19.5005) (-28.8218, 19.5008) (-28.8307, 19.5011) (-28.8396, 19.5014) (-28.8486, 19.5016) (-28.8577, 19.5019) (-28.8668, 19.5021) (-28.8759, 19.5024) (-28.8851, 19.5026) (-28.8943, 19.5028) (-28.9036, 19.503) (-28.9129, 19.5032) (-28.9223, 19.5034) (-28.9317, 19.5036) (-28.9412, 19.5037) (-28.9507, 19.5038) (-28.9602, 19.504) (-28.9698, 19.5041) (-28.9795, 19.5042) (-28.9892, 19.5043) (-28.9989, 19.5043) (-29.0087, 19.5044) (-29.0185, 19.5044) (-29.0284, 19.5045) (-29.0383, 19.5045) (-29.0482, 19.5045) (-29.0582, 19.5045) (-29.0682, 19.5044) (-29.0783, 19.5044) (-29.0884, 19.5043) (-29.0986, 19.5043) (-29.1088, 19.5042) (-29.119, 19.5041) (-29.1293, 19.504) (-29.1396, 19.5038) (-29.15, 19.5037) (-29.1604, 19.5035) (-29.1708, 19.5034) (-29.1813, 19.5032) (-29.1919, 19.503) (-29.2024, 19.5028) (-29.213, 19.5025) (-29.2237, 19.5023) (-29.2344, 19.502) (-29.2451, 19.5017) (-29.2559, 19.5014) (-29.2667, 19.5011) (-29.2775, 19.5008) (-29.2884, 19.5004) (-29.2993, 19.5001) (-29.3103, 19.4997) (-29.3213, 19.4993) (-29.3323, 19.4989) (-29.3434, 19.4984) (-29.3545, 19.498) (-29.3657, 19.4975) (-29.3768, 19.497) (-29.3881, 19.4965) (-29.3993, 19.496) (-29.4106, 19.4955) (-29.422, 19.495) (-29.4333, 19.4944) (-29.4447, 19.4938) (-29.4562, 19.4932) (-29.4677, 19.4926) (-29.4792, 19.492) (-29.4907, 19.4913) (-29.5023, 19.4906) (-29.514, 19.49) (-29.5256, 19.4892) (-29.5373, 19.4885) (-29.549, 19.4878) (-29.5608, 19.487) (-29.5726, 19.4863) (-29.5844, 19.4855) (-29.5963, 19.4846) (-29.6082, 19.4838) (-29.6201, 19.483) (-29.6321, 19.4821) (-29.6441, 19.4812) (-29.6562, 19.4803) (-29.6682, 19.4794) (-29.6803, 19.4784) (-29.6925, 19.4775) (-29.7047, 19.4765) (-29.7169, 19.4755) (-29.7291, 19.4745) (-29.7414, 19.4735) (-29.7537, 19.4724) (-29.766, 19.4713) (-29.7784, 19.4702) (-29.7908, 19.4691) (-29.8032, 19.468) (-29.8157, 19.4669) (-29.8282, 19.4657) (-29.8407, 19.4645) (-29.8533, 19.4633) (-29.8659, 19.4621) (-29.8785, 19.4608) (-29.8912, 19.4596) (-29.9039, 19.4583) (-29.9166, 19.457) (-29.9293, 19.4556) (-29.9421, 19.4543) (-29.9549, 19.4529) (-29.9678, 19.4516) (-29.9806, 19.4501) (-29.9935, 19.4487) (-30.0065, 19.4473) (-30.0194, 19.4458) (-30.0324, 19.4443) (-30.0455, 19.4428) (-30.0585, 19.4413) (-30.0716, 19.4398) (-30.0847, 19.4382) (-30.0979, 19.4366) (-30.111, 19.435) (-30.1242, 19.4334) (-30.1375, 19.4317) (-30.1507, 19.4301) (-30.164, 19.4284) (-30.1773, 19.4267) (-30.1907, 19.425) (-30.2014, 19.4236) (-30.2094, 19.4225) (-30.2148, 19.4218) (-30.2174, 19.4214) knots 0 0 0 0 0 0 0.00416667 0.00833333 0.0125 0.01666667 0.02083333 0.025 0.02916667 0.03333333 0.0375 0.04166667 0.04583333 0.05 0.05416667 0.05833333 0.0625 0.06666667 0.07083333 0.075 0.07916667 0.08333333 0.0875 0.09166667 0.09583333 0.1 0.10416667 0.10833333 0.1125 0.11666667 0.12083333 0.125 0.12916667 0.13333333 0.1375 0.14166667 0.14583333 0.15 0.15416667 0.15833333 0.1625 0.16666667 0.17083333 0.175 0.17916667 0.18333333 0.1875 0.19166667 0.19583333 0.2 0.20416667 0.20833333 0.2125 0.21666667 0.22083333 0.225 0.22916667 0.23333333 0.2375 0.24166667 0.24583333 0.25 0.25416667 0.25833333 0.2625 0.26666667 0.27083333 0.275 0.27916667 0.28333333 0.2875 0.29166667 0.29583333 0.3 0.30416667 0.30833333 0.3125 0.31666667 0.32083333 0.325 0.32916667 0.33333333 0.3375 0.34166667 0.34583333 0.35 0.35416667 0.35833333 0.3625 0.36666667 0.37083333 0.375 0.37916667 0.38333333 0.3875 0.39166667 0.39583333 0.4 0.40416667 0.40833333 0.4125 0.41666667 0.42083333 0.425 0.42916667 0.43333333 0.4375 0.44166667 0.44583333 0.45 0.45416667 0.45833333 0.4625 0.46666667 0.47083333 0.475 0.47916667 0.48333333 0.4875 0.49166667 0.49583333 0.5 0.50416667 0.50833333 0.5125 0.51666667 0.52083333 0.525 0.52916667 0.53333333 0.5375 0.54166667 0.54583333 0.55 0.55416667 0.55833333 0.5625 0.56666667 0.57083333 0.575 0.57916667 0.58333333 0.5875 0.59166667 0.59583333 0.6 0.60416667 0.60833333 0.6125 0.61666667 0.62083333 0.625 0.62916667 0.63333333 0.6375 0.64166667 0.64583333 0.65 0.65416667 0.65833333 0.6625 0.66666667 0.67083333 0.675 0.67916667 0.68333333 0.6875 0.69166667 0.69583333 0.7 0.70416667 0.70833333 0.7125 0.71666667 0.72083333 0.725 0.72916667 0.73333333 0.7375 0.74166667 0.74583333 0.75 0.75416667 0.75833333 0.7625 0.76666667 0.77083333 0.775 0.77916667 0.78333333 0.7875 0.79166667 0.79583333 0.8 0.80416667 0.80833333 0.8125 0.81666667 0.82083333 0.825 0.82916667 0.83333333 0.8375 0.84166667 0.84583333 0.85 0.85416667 0.85833333 0.8625 0.86666667 0.87083333 0.875 0.87916667 0.88333333 0.8875 0.89166667 0.89583333 0.9 0.90416667 0.90833333 0.9125 0.91666667 0.92083333 0.925 0.92916667 0.93333333 0.9375 0.94166667 0.94583333 0.95 0.95416667 0.95833333 0.9625 0.96666667 0.97083333 0.975 0.97916667 0.98333333 0.9875 0.99166667 0.99583333 1 1 1 1 1 1
  line L235 (-28.7355, 13.4119) -> (-29.0298, 13.4213)
  spline S106 degree 5 poles (21.1029, -10.2084) (21.1018, -10.2059) (21.0998, -10.2009) (21.0967, -10.1934) (21.0925, -10.1834) (21.0873, -10.171) (21.0822, -10.1586) (21.077, -10.1462) (21.0718, -10.1339) (21.0666, -10.1217) (21.0614, -10.1094) (21.0562, -10.0972) (21.051, -10.085) (21.0458, -10.0729) (21.0406, -10.0608) (21.0354, -10.0487) (21.0302, -10.0367) (21.025, -10.0247) (21.0198, -10.0127) (21.0145, -10.0008) (21.0093, -9.9889) (21.0041, -9.9771) (20.9989, -9.9653) (20.9937, -9.9535) (20.9884, -9.9417) (20.9832, -9.93) (20.978, -9.9184) (20.9727, -9.9067) (20.9675, -9.8951) (20.9623, -9.8836) (20.957, -9.8721) (20.9518, -9.8606) (20.9466, -9.8491) (20.9413, -9.8377) (20.9361, -9.8264) (20.9308, -9.815) (20.9256, -9.8037) (20.9204, -9.7925) (20.9151, -9.7812) (20.9099, -9.7701) (20.9046, -9.7589) (20.8994, -9.7478) (20.8942, -9.7367) (20.8889, -9.7257) (20.8837, -9.7147) (20.8784, -9.7038) (20.8732, -9.6928) (20.868, -9.682) (20.8627, -9.6711) (20.8575, -9.6603) (20.8523, -9.6496) (20.847, -9.6388) (20.8418, -9.6281) (20.8366, -9.6175) (20.8313, -9.6069) (20.8261, -9.5963) (20.8209, -9.5858) (20.8157, -9.5753) (20.8105, -9.5649) (20.8052, -9.5544) (20.8, -9.5441) (20.7948, -9.5337) (20.7896, -9.5235) (20.7844, -9.5132) (20.7792, -9.503) (20.774, -9.4928) (20.7688, -9.4827) (20.7636, -9.4726) (20.7584, -9.4625) (20.7532, -9.4525) (20.748, -9.4426) (20.7429, -9.4326) (20.7377, -9.4228) (20.7325, -9.4129) (20.7274, -9.4031) (20.7222, -9.3933) (20.717, -9.3836) (20.7119, -9.3739) (20.7067, -9.3643) (20.7016, -9.3547) (20.6965, -9.3451) (20.6913, -9.3356) (20.6862, -9.3261) (20.6811, -9.3167) (20.676, -9.3073) (20.6709, -9.298) (20.6658, -9.2887) (20.6607, -9.2794) (20.6556, -9.2702) (20.6505, -9.261) (20.6454, -9.2519) (20.6404, -9.2428) (20.6353, -9.2337) (20.6303, -9.2247) (20.6252, -9.2158) (20.6202, -9.2068) (20.6152, -9.198) (20.6101, -9.1891) (20.6051, -9.1803) (20.6001, -9.1716) (20.5951, -9.1629) (20.5902, -9.1542) (20.5852, -9.1456) (20.5802, -9.1371) (20.5753, -9.1285) (20.5703, -9.1201) (20.5654, -9.1116) (20.5605, -9.1032) (20.5555, -9.0949) (20.5506, -9.0866) (20.5457, -9.0783) (20.5409, -9.0701) (20.536, -9.0619) (20.5311, -9.0538) (20.5263, -9.0458) (20.5214, -9.0377) (20.5166, -9.0297) (20.5118, -9.0218) (20.507, -9.0139) (20.5022, -9.0061) (20.4974, -8.9983) (20.4927, -8.9905) (20.4879, -8.9828) (20.4832, -8.9752) (20.4784, -8.9676) (20.4737, -8.96) (20.469, -8.9525) (20.4644, -8.945) (20.4597, -8.9376) (20.455, -8.9302) (20.4504, -8.9229) (20.4458, -8.9156) (20.4412, -8.9084) (20.4366, -8.9012) (20.432, -8.8941) (20.4274, -8.887) (20.4229, -8.88) (20.4184, -8.873) (20.4139, -8.8661) (20.4094, -8.8592) (20.4049, -8.8523) (20.4004, -8.8455) (20.396, -8.8388) (20.3916, -8.8321) (20.3872, -8.8255) (20.3828, -8.8189) (20.3784, -8.8124) (20.3741, -8.8059) (20.3698, -8.7995) (20.3655, -8.7931) (20.3612, -8.7867) (20.3569, -8.7805) (20.3527, -8.7742) (20.3484, -8.7681) (20.3442, -8.7619) (20.3401, -8.7559) (20.3359, -8.7498) (20.3318, -8.7439) (20.3277, -8.738) (20.3236, -8.7321) (20.3195, -8.7263) (20.3155, -8.7205) (20.3115, -8.7148) (20.3075, -8.7092) (20.3035, -8.7036) (20.2996, -8.6981) (20.2956, -8.6926) (20.2918, -8.6871) (20.2879, -8.6818) (20.2841, -8.6764) (20.2802, -8.6712) (20.2765, -8.666) (20.2727, -8.6608) (20.269, -8.6557) (20.2653, -8.6507) (20.2616, -8.6457) (20.258, -8.6408) (20.2544, -8.6359) (20.2508, -8.6311) (20.2472, -8.6263) (20.2437, -8.6216) (20.2402, -8.617) (20.2368, -8.6124) (20.2333, -8.6079) (20.23, -8.6034) (20.2266, -8.599) (20.2233, -8.5947) (20.22, -8.5904) (20.2167, -8.5862) (20.2135, -8.582) (20.2103, -8.5779) (20.2072, -8.5739) (20.2041, -8.5699) (20.201, -8.566) (20.198, -8.5621) (20.195, -8.5583) (20.192, -8.5546) (20.1891, -8.5509) (20.1862, -8.5473) (20.1834, -8.5437) (20.1806, -8.5403) (20.1778, -8.5368) (20.1751, -8.5335) (20.1724, -8.5302) (20.1698, -8.527) (20.1672, -8.5238) (20.1647, -8.5207) (20.1622, -8.5177) (20.1597, -8.5148) (20.1573, -8.5119) (20.155, -8.509) (20.1527, -8.5063) (20.1504, -8.5036) (20.1482, -8.501) (20.1461, -8.4984) (20.144, -8.496) (20.1419, -8.4936) (20.1399, -8.4912) (20.138, -8.489) (20.1361, -8.4868) (20.1343, -8.4847) (20.1325, -8.4826) (20.1308, -8.4806) (20.1291, -8.4787) (20.1275, -8.4769) (20.126, -8.4752) (20.1245, -8.4735) (20.123, -8.4719) (20.1217, -8.4704) (20.1204, -8.4689) (20.1192, -8.4675) (20.118, -8.4663) (20.1169, -8.4651) (20.1159, -8.4639) (20.1149, -8.4629) (20.114, -8.4619) (20.1132, -8.461) (20.1125, -8.4602) (20.1118, -8.4595) (20.1112, -8.4589) (20.1107, -8.4583) (20.1104, -8.458) (20.1102, -8.4577) (20.11, -8.4576) (20.11, -8.4575) knots -1 -1 -1 -1 -1 -1 -0.99583333 -0.99166667 -0.9875 -0.98333333 -0.97916667 -0.975 -0.97083333 -0.96666667 -0.9625 -0.95833333 -0.95416667 -0.95 -0.94583333 -0.94166667 -0.9375 -0.93333333 -0.92916667 -0.925 -0.92083333 -0.91666667 -0.9125 -0.90833333 -0.90416667 -0.9 -0.89583333 -0.89166667 -0.8875 -0.88333333 -0.87916667 -0.875 -0.87083333 -0.86666667 -0.8625 -0.85833333 -0.85416667 -0.85 -0.84583333 -0.84166667 -0.8375 -0.83333333 -0.82916667 -0.825 -0.82083333 -0.81666667 -0.8125 -0.80833333 -0.80416667 -0.8 -0.79583333 -0.79166667 -0.7875 -0.78333333 -0.77916667 -0.775 -0.77083333 -0.76666667 -0.7625 -0.75833333 -0.75416667 -0.75 -0.74583333 -0.74166667 -0.7375 -0.73333333 -0.72916667 -0.725 -0.72083333 -0.71666667 -0.7125 -0.70833333 -0.70416667 -0.7 -0.69583333 -0.69166667 -0.6875 -0.68333333 -0.67916667 -0.675 -0.67083333 -0.66666667 -0.6625 -0.65833333 -0.65416667 -0.65 -0.64583333 -0.64166667 -0.6375 -0.63333333 -0.62916667 -0.625 -0.62083333 -0.61666667 -0.6125 -0.60833333 -0.60416667 -0.6 -0.59583333 -0.59166667 -0.5875 -0.58333333 -0.57916667 -0.575 -0.57083333 -0.56666667 -0.5625 -0.55833333 -0.55416667 -0.55 -0.54583333 -0.54166667 -0.5375 -0.53333333 -0.52916667 -0.525 -0.52083333 -0.51666667 -0.5125 -0.50833333 -0.50416667 -0.5 -0.49583333 -0.49166667 -0.4875 -0.48333333 -0.47916667 -0.475 -0.47083333 -0.46666667 -0.4625 -0.45833333 -0.45416667 -0.45 -0.44583333 -0.44166667 -0.4375 -0.43333333 -0.42916667 -0.425 -0.42083333 -0.41666667 -0.4125 -0.40833333 -0.40416667 -0.4 -0.39583333 -0.39166667 -0.3875 -0.38333333 -0.37916667 -0.375 -0.37083333 -0.36666667 -0.3625 -0.35833333 -0.35416667 -0.35 -0.34583333 -0.34166667 -0.3375 -0.33333333 -0.32916667 -0.325 -0.32083333 -0.31666667 -0.3125 -0.30833333 -0.30416667 -0.3 -0.29583333 -0.29166667 -0.2875 -0.28333333 -0.27916667 -0.275 -0.27083333 -0.26666667 -0.2625 -0.25833333 -0.25416667 -0.25 -0.24583333 -0.24166667 -0.2375 -0.23333333 -0.22916667 -0.225 -0.22083333 -0.21666667 -0.2125 -0.20833333 -0.20416667 -0.2 -0.19583333 -0.19166667 -0.1875 -0.18333333 -0.17916667 -0.175 -0.17083333 -0.16666667 -0.1625 -0.15833333 -0.15416667 -0.15 -0.14583333 -0.14166667 -0.1375 -0.13333333 -0.12916667 -0.125 -0.12083333 -0.11666667 -0.1125 -0.10833333 -0.10416667 -0.1 -0.09583333 -0.09166667 -0.0875 -0.08333333 -0.07916667 -0.075 -0.07083333 -0.06666667 -0.0625 -0.05833333 -0.05416667 -0.05 -0.04583333 -0.04166667 -0.0375 -0.03333333 -0.02916667 -0.025 -0.02083333 -0.01666667 -0.0125 -0.00833333 -0.00416667 0 0 0 0 0 0
  arc A117 (23.3609, 32.8781) -> (22.7084, 33.6029) centre (0, 12.5) ccw
  arc A118 (-29.6298, 3.3854) -> (-29.3284, 2.4579) centre (0, 12.5) ccw